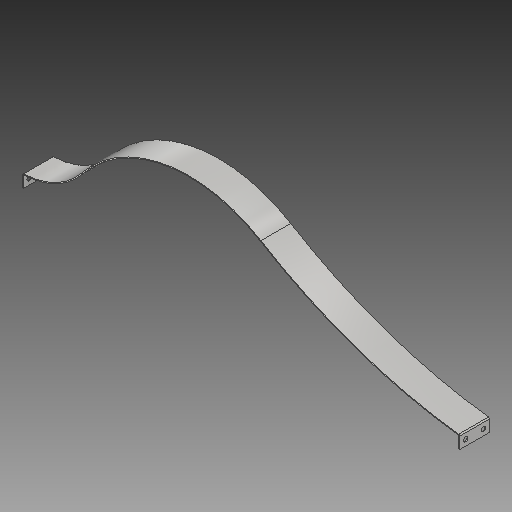
# Autodesk Inventor part: 8inch_Fin
Saved by Autodesk Inventor 2017 (Build 210142000, 142)
## iProperties
Created: 2016-05-03
Part Number: 8inch_Fin
Material: Generic
Document SubType Name: Modeling
Designer: Andres
Density: 1 g/cm^3
Appearance: Aluminum - Polished
Mass: 7.97267 g
Surface Area: 217.034 cm^2
Volume: 7.97267 cm^3
Author: Andres
Autodesk Inventor part; units mm, degrees
ref_plane "YZ Plane" through (0, 0, 0) normal (1, 0, 0) x (0, 1, 0)
ref_plane "XZ Plane" through (0, 0, 0) normal (0, 1, 0) x (-1, 0, 0)
ref_plane "XY Plane" through (0, 0, 0) normal (0, 0, 1) x (1, 0, 0)
sketch "Sketch1" plane through (0, 0, 0) normal (0, 0, 1) x (1, 0, 0)
  line L0 (0, 0) -> (150, 0)
  line L1 (150, 0) -> (150, 68)
  line L2 (150, 68) -> (0, 68)
  line L3 (0, 68) -> (0, 0)
  arc A0 (150, 51.1345) -> (0, 24.6854) centre (90, -47.1593) ccw
  line L4 (0, 24.6854) -> (150, 51.1345) construction
  line L5 (0, 24.6854) -> (152.314, 24.6854) construction
  arc A1 (-49, -0.0229) -> (0, 24.6854) centre (-51.433, 65.743) ccw
  arc A2 (150, 51.1345) -> (316.5, -6.6745) centre (366.3369, 405.5438) ccw
  arc A3 (150.396, 51.7832) -> (317.26, -6.0003) centre (366.3369, 405.5438) ccw
  arc A4 (150.396, 51.7832) -> (-0.594, 25.1596) centre (90, -47.1593) ccw
  arc A5 (-48.9969, 0.7377) -> (-0.594, 25.1596) centre (-51.433, 65.743) ccw
  line L6 (-49, -0.0229) -> (-49, -10.0229)
  line L7 (-49, -10.0229) -> (-49.76, -10.0229)
  line L8 (-49.76, -10.0229) -> (-49.76, 0.7377)
  line L9 (-49.76, 0.7377) -> (-48.9969, 0.7377)
  line L10 (316.5, -6.6745) -> (316.5, -16.6745)
  line L11 (316.5, -16.6745) -> (317.26, -16.6745)
  line L12 (317.26, -16.6745) -> (317.26, -6.0003)
  line L13 (317.26, -6.0003) -> (317.26, -6.0003)
  dimension "d0" = 150
  dimension "d1" = 68
  dimension "d2" = 10
  dimension "d3" = 90
  dimension "d4" = 65.8109
  dimension "d5" = 49
  dimension "d6" = 415.22
  dimension "d7" = 166.5
  dimension "d10" = 0.76
  dimension "d56" = 10
  dimension "d57" = 0.76
  dimension "d59" = 10
  dimension "d60" = 0.76
  dimension "d61" = 90
  constraints: 28 end point, 13 point on circle, 6 centre point, 5 perpendicular, 3 horizontal, 3 tangent, 2 parallel, 2 point on line, 2 vertical, 1 equal length, 2 other
  measures "d0" distance of L1.end L2.end
  measures "d1" distance of L0.end L1.end
  measures "d2" angle of L5 L4
  measures "d3" horizontal distance of A0.centre L4.start
  measures "d4" radius of A1
  measures "d5" distance of L0.start L6.start
  measures "d6" radius of A2
  measures "d7" distance from line of L10.start L1
  measures "d10" radial gap between concentric circles of A1 A5
  measures "d56" distance of L6.start L6.end
  measures "d57" distance of L6.end L7.end
  measures "d59" distance of L10.start L10.end
  measures "d60" distance of L10.end L11.end
  measures "d61" angle of L12 L11
extrude "Extrusion1" add sketch "Sketch1" along normal blind 25 contours A1 L6 L7 L8 L9 A5 A4 L3 | L3 A4 L2 A0 | A0 L2 A4 L1 | L1 A4 A3 L12 L11 L10 A2 | L2 A4
fillet "Fillet1" radius 6 1 edges at (-48.9969, 0.7377, 12.5)
fillet "Fillet2" radius 1 1 edges at (-49.76, 0.7377, 12.5)
fillet "Fillet3" radius 1 1 edges at (317.26, -6.0003, 12.5)
ref_plane "Work Plane1" through (317.26, -16.6745, 25) normal (1, 0, 0) x (0, 0, -1)
sketch "Sketch8" plane through (317.26, -16.6745, 25) normal (1, 0, 0) x (0, 0, -1)
  line L0 (0, 9.7873) -> (25, 9.7873) projected
  line L1 (0, 0) -> (0, 9.7873) projected
  line L2 (25, 0) -> (0, 0) projected
  line L3 (25, 0) -> (25, 9.7873) projected
  point P0 (25, 16.6745)
  point P1 (5, 5)
  point P2 (20, 5)
  dimension "d65" = 5
  dimension "d66" = 5
  dimension "d68" = 5
  dimension "d69" = 5
  measures "d65" distance from line of L3 point (20, 5)
  measures "d66" distance from line of L1 point (5, 5)
  measures "d68" distance from line of L2 point (5, 5)
  measures "d69" distance from line of L2 point (20, 5)
ref_plane "Work Plane2" through (-49.76, -10.0229, 0) normal (-1, 0, 0) x (0, 0, 1)
sketch "Sketch9" plane through (-49.76, -10.0229, 0) normal (-1, 0, 0) x (0, 0, 1)
  line L0 (0, 9.7691) -> (25, 9.7691) projected
  line L1 (0, 9.7691) -> (0, 0) projected
  line L2 (0, 0) -> (25, 0) projected
  line L3 (25, 9.7691) -> (25, 0) projected
  point P0 (0, 10.0229)
  point P1 (5, 5)
  point P2 (20, 5)
  dimension "d71" = 5
  dimension "d72" = 5
  dimension "d73" = 5
  dimension "d74" = 5
  measures "d71" distance from line of L2 point (20, 5)
  measures "d72" distance from line of L2 point (5, 5)
  measures "d73" distance from line of L3 point (20, 5)
  measures "d74" distance from line of point (5, 5) L1
hole "Hole3" at (-49.76, -5.0229, 20) at (-49.76, -5.0229, 5) direction (1, 0, 0) diameter 4 depth 0.76
hole "Hole4" at (317.26, -11.6745, 20) at (317.26, -11.6745, 5) direction (-1, 0, 0) diameter 4 depth 0.76
body "Solid1"
